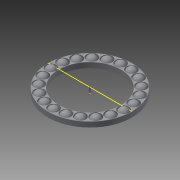
# Autodesk Inventor part: ThrustBearing-GuideRingCage
Saved by Autodesk Inventor 2015 (Build 190159000, 159)
## iProperties
Created: 2014-04-13
Part Number: ThrustBearing-GuideRingCage
Material: Generic
Document SubType Name: Modeling
Designer: Will Stuckey
Density: 1 g/cm^3
Appearance: Default
Author: Will Stuckey
Autodesk Inventor part; units mm, degrees
ref_plane "YZ Plane" through (0, 0, 0) normal (1, 0, 0) x (0, 1, 0)
ref_plane "XZ Plane" through (0, 0, 0) normal (0, 1, 0) x (-1, 0, 0)
ref_plane "XY Plane" through (0, 0, 0) normal (0, 0, 1) x (1, 0, 0)
sketch "Sketch1" plane through (0, 0, 0) normal (0, 1, 0) x (-1, 0, 0)
  circle A0 centre (0, 0) radius 25.4
  circle A1 centre (0, 0) radius 18.6531
  dimension "d0" = 50.8
  dimension "d1" = 37.3062
  constraints: 2 centre point, 2 coincident
  measures "d0" diameter of A0
  measures "d1" diameter of A1
extrude "Extrusion1" add sketch "Sketch1" along normal blind 3.175
sketch "Sketch2" plane through (0, 0, 0) normal (1, 0, 0) x (0, 1, 0)
  point P0 (0, 0)
sketch "Sketch3" plane through (0, 0, 0) normal (0, 1, 0) x (-1, 0, 0)
  circle A0 centre (0, 22.0266) radius 2.7781
  point P0 (0, 0)
  dimension "d4" = 5.5563
  constraints: 1 centre point
  measures "d4" diameter of A0
sketch "Sketch4" plane through (0, 0, 0) normal (0, 0, 1) x (1, 0, 0)
  line L0 (0, 0) -> (0, 3.175)
  line L1 (25.4, 3.175) -> (-25.4, 3.175) projected
  constraints: 2 end point, 1 midpoint
hole "Hole1" at (0, 0, 22.0266) direction (0, 1, 0) diameter 6.35 depth 3.175 tip angle 118
pattern_circular "Circular Pattern1" count 21 over 360 about axis through (0, 0, 0) along (0, 1, 0) of "Hole1"
sketch "Sketch5" plane through (0, 0, 0) normal (1, 0, 0) x (0, 1, 0)
  line L0 (0, 25.4) -> (0, -25.4) projected
  line L1 (0, -19.4469) -> (2.7781, -19.2484)
  line L2 (0, -19.4469) -> (2.7852, -19.4469) construction
  line L3 (0, -24.6062) -> (2.7781, -24.8047)
  line L4 (0, -24.6062) -> (2.7852, -24.6062) construction
  line L5 (2.7781, -24.8047) -> (2.7781, -19.2484)
  line L6 (3.175, -25.4) -> (3.175, 25.4) projected
  line L7 (0, -24.6062) -> (0, -19.4469)
  line L8 (0, 0) -> (3.175, 0)
  dimension "d15" = 2.7852
  dimension "d16" = 4.086
  dimension "d17" = 2.7852
  dimension "d18" = 4.086
  constraints: 14 end point, 2 equal length, 2 horizontal, 1 midpoint, 1 parallel, 1 point on line
  measures "d15" distance of L1.start L1.end
  measures "d16" angle of L2 L1
  measures "d17" distance of L3.start L3.end
  measures "d18" angle of L3 L4
revolve "Revolution1" cut sketch "Sketch5" angle 360 about axis through (0, 0, 0) along (0, 1, 0)
fillet "Fillet1" radius 0.1984 1 edges at (25.4, 3.175, 0)
fillet "Fillet2" radius 0.1984 1 edges at (18.6531, 3.175, 0)
sketch "Sketch6" plane through (0, 0, 0) normal (1, 0, 0) x (0, 1, 0)
  line L0 (-1.0914, 22.0266) -> (4.4648, 22.0266)
  line L1 (-1.0914, 22.0266) -> (4.4648, 22.0266) construction
  arc A0 (-1.0914, 22.0266) -> (4.4648, 22.0266) centre (1.6867, 21.8865) ccw
  line L2 (4.4648, 22.0266) -> (-1.0914, 22.0266)
  point P0 (0, 0)
  dimension "d22" = 5.5563
  dimension "d23" = 0
  constraints: 6 end point, 3 horizontal, 2 point on circle, 1 centre point, 1 collinear
  measures "d22" distance of L0.start L0.end
  measures "d23" distance between parallel lines of L0 L1
revolve "Revolution2" add sketch "Sketch6" angle 360 about axis through (0, -1.0914, 22.0266) along (0, 1, 0)
pattern_circular "Circular Pattern2" count 21 over 360 about axis through (0, 0, 0) along (0, 1, 0) of "Revolution2"
body "Solid1"
